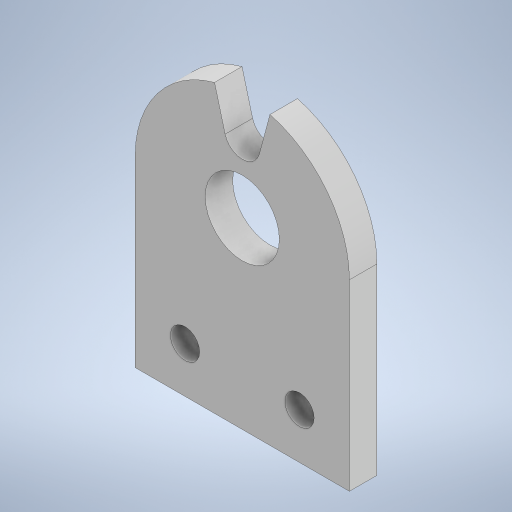
# Autodesk Inventor part: Xgantry_CableChain_top_connector
Saved by Autodesk Inventor 2023 (Build 270158000, 158)
## iProperties
Created: 2023-01-08
Part Number: Xgantry_CableChain_top_connector
Material: Generic
Document SubType Name: Modeling
Designer: a laptop
Density: 1 g/cm^3
Appearance: Default
Author: a laptop
Autodesk Inventor part; units mm, degrees
ref_plane "YZ Plane" through (0, 0, 0) normal (1, 0, 0) x (0, 1, 0)
ref_plane "XZ Plane" through (0, 0, 0) normal (0, 1, 0) x (-1, 0, 0)
ref_plane "XY Plane" through (0, 0, 0) normal (0, 0, 1) x (1, 0, 0)
sketch "Sketch1" plane through (0, 0, 0) normal (0, 0, 1) x (1, 0, 0)
  arc A0 (-1.9, 11.5447) -> (-3.0282, 11.3013) centre (0, 0) ccw construction
  line L0 (0, 7.75) -> (0, 0) construction
  arc A1 (1.9, 11.5447) -> (-1.9, 11.5447) centre (0, 0) ccw construction
  circle A2 centre (0, 0) radius 4.05
  line L1 (11.7, 0) -> (11.7, -20)
  line L2 (11.7, -20) -> (-11.7, -20)
  line L3 (-11.7, -20) -> (-11.7, 0)
  arc A3 (11.7, 0) -> (3.0282, 11.3013) centre (0, 0) ccw
  arc A4 (-11.7, 0) -> (11.7, 0) centre (0, 0) ccw construction
  line L4 (3.0282, 11.3013) -> (1.872, 6.9864)
  line L5 (-1.872, 6.9864) -> (-3.0282, 11.3013)
  arc A5 (-1.872, 6.9864) -> (1.872, 6.9864) centre (0, 7.488) ccw
  arc A6 (3.0282, 11.3013) -> (1.9, 11.5447) centre (0, 0) ccw construction
  arc A7 (-3.0282, 11.3013) -> (-11.7, 0) centre (0, 0) ccw
  line L6 (-1.872, 6.9864) -> (0, 0) construction
  line L7 (0, 0) -> (1.872, 6.9864) construction
  line L8 (0, 5.55) -> (0, 4.05) construction
  dimension "d3" = 8.1
  dimension "d0" = 23.4
  dimension "d4" = 20
  dimension "d8" = 30
  dimension "d9" = 1.5
  constraints: 18 end point, 17 point on circle, 7 centre point, 6 tangent, 3 coincident, 3 vertical, 2 collinear, 1 horizontal alignment, 1 parallel, 1 perpendicular, 1 point on line, 1 vertical alignment, 2 other
  measures "d0" diameter of A0
  measures "d4" distance from line of L2 point (0, 0)
  measures "d8" angle of L4 L5
  measures "d9" distance of L8.start L8.end
extrude "Extrusion1" add sketch "Sketch1" along normal blind 3
sketch "Sketch2" plane through (0, 0, 3) normal (0, 0, 1) x (1, 0, 0)
  circle A0 centre (-6.25, -15) radius 1.6
  circle A1 centre (6.25, -15) radius 1.6
  line L0 (-6.25, -15) -> (6.25, -15) construction
  line L1 (0, -15) -> (0, -20) construction
  line L2 (-11.7, -20) -> (11.7, -20) construction
  point P0 (0, 0)
  dimension "d10" = 3.2
  dimension "d11" = 5
  dimension "d12" = 12.5
  constraints: 4 end point, 2 centre point, 2 midpoint, 1 coincident, 1 equal radius, 1 horizontal, 1 perpendicular
  measures "d10" diameter of A0
  measures "d11" distance of L1.start L1.end
  measures "d12" distance of L0.start L0.end
extrude "Extrusion2" cut sketch "Sketch2" against normal through all
body "Solid1"
